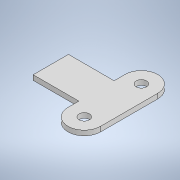
# Autodesk Inventor part: Проставка для двигателя
Saved by Autodesk Inventor 2020 (Build 240168000, 168)
## iProperties
Created: 2021-06-02
Part Number: Проставка для двигателя
Material: Типовые
Document SubType Name: Modeling
Designer: Антон
Density: 1 g/cm^3
Appearance: По умолчанию
Author: Антон
Autodesk Inventor part; units mm, degrees
ref_plane "YZ Plane" through (0, 0, 0) normal (1, 0, 0) x (0, 1, 0)
ref_plane "XZ Plane" through (0, 0, 0) normal (0, 1, 0) x (-1, 0, 0)
ref_plane "XY Plane" through (0, 0, 0) normal (0, 0, 1) x (1, 0, 0)
sketch "Эскиз1" plane through (0, 0, 0) normal (0, 1, 0) x (-1, 0, 0)
  line L0 (0, 0) -> (0, -17.5) construction
  line L1 (-5, 0) -> (-5, -17.5)
  line L2 (5, -17.5) -> (5, 0)
  arc A0 (5, 0) -> (-5, 0) centre (0, 0) ccw
  arc A1 (-5, -17.5) -> (5, -17.5) centre (0, -17.5) ccw
  line L3 (5, -14.15) -> (19, -14.15)
  line L4 (19, -14.15) -> (19, -3.35)
  line L5 (19, -3.35) -> (5, -3.35)
  line L6 (5, -3.35) -> (5, -14.15)
  circle A2 centre (0, 0) radius 1.6
  circle A3 centre (0, -17.5) radius 1.6
  point P0 (0, -8.75)
  point P1 (5, -8.75)
  dimension "d0" = 17.5
  dimension "d1" = 5
  dimension "d3" = 24
  dimension "d4" = 10.8
  dimension "d5" = 3.2
  constraints: 16 end point, 4 centre point, 4 point on circle, 4 tangent, 3 midpoint, 3 parallel, 2 coincident, 1 equal radius, 1 horizontal, 1 perpendicular, 1 vertical
  measures "d0" distance of L0.start L0.end
  measures "d1" radius of A1
  measures "d3" distance between parallel lines of L1 L4
  measures "d4" distance of L3.end L4.end
  measures "d5" diameter of A2
extrude "Выдавливание1" add sketch "Эскиз1" along normal blind 1.5
